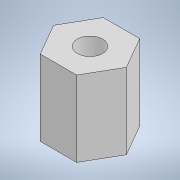
# Autodesk Inventor part: Проставка для стойки RPLIDAR
Saved by Autodesk Inventor 2020 (Build 240168000, 168)
## iProperties
Created: 2021-07-27
Part Number: Проставка для стойки RPLIDAR
Material: Типовые
Document SubType Name: Modeling
Designer: Антон
Density: 1 g/cm^3
Appearance: По умолчанию
Author: Антон
Autodesk Inventor part; units mm, degrees
ref_plane "YZ Plane" through (0, 0, 0) normal (1, 0, 0) x (0, 1, 0)
ref_plane "XZ Plane" through (0, 0, 0) normal (0, 1, 0) x (-1, 0, 0)
ref_plane "XY Plane" through (0, 0, 0) normal (0, 0, 1) x (1, 0, 0)
sketch "Эскиз1" plane through (0, 0, 0) normal (0, 1, 0) x (-1, 0, 0)
  line L0 (1.4434, 2.5) -> (2.8868, 0)
  line L1 (2.8868, 0) -> (1.4434, -2.5)
  line L2 (1.4434, -2.5) -> (-1.4434, -2.5)
  line L3 (-1.4434, -2.5) -> (-2.8868, 0)
  line L4 (-2.8868, 0) -> (-1.4434, 2.5)
  line L5 (-1.4434, 2.5) -> (1.4434, 2.5)
  point P0 (0, 0)
  point P1 (0, 0)
  dimension "d0" = 5
  constraints: 12 end point, 1 coincident, 1 horizontal, 13 other
  measures "d0" distance between parallel lines of L2 L5
extrude "Выдавливание1" add sketch "Эскиз1" along normal blind 6
sketch "Эскиз2" plane through (0, 6, 0) normal (0, 1, 0) x (1, 0, 0)
  line L0 (1.4434, 2.5) -> (-1.4434, 2.5) projected
  line L1 (-1.4434, 2.5) -> (-2.8868, 0) projected
  line L2 (-2.8868, 0) -> (-1.4434, -2.5) projected
  line L3 (-1.4434, -2.5) -> (1.4434, -2.5) projected
  line L4 (1.4434, -2.5) -> (2.8868, 0) projected
  line L5 (2.8868, 0) -> (1.4434, 2.5) projected
  point P0 (0, 0)
hole "Отверстие1" at (0, 6, 0) direction (0, -1, 0) diameter 2 end through all
